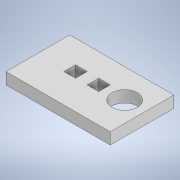
# Autodesk Inventor part: RCcar_motor_testplate
Saved by Autodesk Inventor 2022 (Build 260153000, 153)
## iProperties
Created: 2022-03-25
Part Number: RCcar_motor_testplate
Material: Generic
Document SubType Name: Modeling
Designer: saipr
Density: 1 g/cm^3
Appearance: Default
Author: saipr
Autodesk Inventor part; units mm, degrees
ref_plane "YZ Plane" through (0, 0, 0) normal (1, 0, 0) x (0, 1, 0)
ref_plane "XZ Plane" through (0, 0, 0) normal (0, 1, 0) x (-1, 0, 0)
ref_plane "XY Plane" through (0, 0, 0) normal (0, 0, 1) x (1, 0, 0)
sketch "Sketch1" plane through (0, 0, 0) normal (0, 1, 0) x (-1, 0, 0)
  line L0 (57.15, 34.925) -> (57.15, 0)
  line L1 (57.15, 34.925) -> (0, 34.925)
  line L2 (57.15, 0) -> (57.15, 15.875)
  line L3 (34.925, 12.7) -> (41.275, 12.7)
  line L4 (41.275, 12.7) -> (41.275, 19.05)
  line L5 (41.275, 19.05) -> (34.925, 19.05)
  line L6 (34.925, 19.05) -> (34.925, 12.7)
  line L7 (34.925, 12.7) -> (41.275, 19.05) construction
  line L8 (41.275, 12.7) -> (34.925, 19.05) construction
  line L9 (28.575, 12.7) -> (22.225, 12.7)
  line L10 (22.225, 12.7) -> (22.225, 19.05)
  line L11 (22.225, 19.05) -> (28.575, 19.05)
  line L12 (28.575, 19.05) -> (28.575, 12.7)
  line L13 (28.575, 12.7) -> (22.225, 19.05) construction
  line L14 (22.225, 12.7) -> (28.575, 19.05) construction
  circle A0 centre (11.1125, 15.875) radius 6.985
  line L15 (57.15, 34.925) -> (3.175, 34.925)
  line L16 (3.175, 0) -> (57.15, 0)
  line L17 (57.15, 0) -> (57.15, 34.925)
  line L18 (0, 34.925) -> (0, 0)
  line L19 (0, 0) -> (57.15, 0)
  point P0 (0, 0)
  dimension "d0" = 57.15
  dimension "d1" = 15.875
  dimension "d4" = 6.35
  dimension "d5" = 6.35
  dimension "d6" = 6.35
  dimension "d7" = 6.35
  dimension "d9" = 13.97
  dimension "d11" = 0
  dimension "d12" = 53.975
  dimension "d13" = 57.15
  dimension "d14" = 34.925
  dimension "d15" = 90
  dimension "d16" = 3.175
  dimension "d17" = 12.7
  dimension "d18" = 12.7
  dimension "d19" = 6.35
  dimension "d20" = 15.875
  dimension "d21" = 11.1125
  dimension "d22" = 15.875
  dimension "d23" = 11.1125
  dimension "d24" = 34.925
  constraints: 40 end point, 5 parallel, 4 horizontal, 2 perpendicular, 1 centre point, 1 collinear, 1 point on line, 1 vertical
  measures "d0" distance of L0.start L1.end
  measures "d1" distance of L2.start L2.end
  measures "d4" distance of L6.start L7.end
  measures "d5" distance of L7.end L3.end
  measures "d6" distance of L10.end L12.start
  measures "d7" distance of L9.end L10.end
  measures "d9" diameter of A0
  measures "d11" distance from line of point (0, 0) L18
  measures "d12" distance of L16.start L16.end
  measures "d13" distance of L18.end L16.end
  measures "d14" distance of L0.start L2.start
  measures "d15" angle of L0 L1
  measures "d16" distance from line of L18 L15.end
  measures "d17" distance between parallel lines of L16 L9
  measures "d18" distance between parallel lines of L16 L3
  measures "d19" distance from line of L6.start L12
  measures "d20" distance from line of L16 A0.centre
  measures "d21" distance from line of L18 A0.centre
  measures "d22" distance from line of L1 L7.end
  measures "d23" horizontal distance of L10.end A0.centre
  measures "d24" distance from line of point (0, 0) L15
extrude "Extrusion1" add sketch "Sketch1" along normal blind 6.35
body "Solid1"
